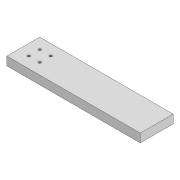
# Autodesk Inventor part: theplank
Saved by Autodesk Inventor 2020 (Build 240168000, 168)
## iProperties
Created: 2021-06-21
Part Number: theplank
Material: Generic
Document SubType Name: Modeling
Designer: Aidan Lee
Density: 1 g/cm^3
Appearance: Default
Author: Aidan Lee
Autodesk Inventor part; units mm, degrees
ref_plane "YZ Plane" through (0, 0, 0) normal (1, 0, 0) x (0, 1, 0)
ref_plane "XZ Plane" through (0, 0, 0) normal (0, 1, 0) x (-1, 0, 0)
ref_plane "XY Plane" through (0, 0, 0) normal (0, 0, 1) x (1, 0, 0)
sketch "Sketch1" plane through (0, 0, 0) normal (0, 1, 0) x (-1, 0, 0)
  line L0 (0, 0) -> (-280, 0)
  line L1 (-280, 0) -> (-280, -69)
  line L2 (-280, -69) -> (0, -69)
  line L3 (0, -69) -> (0, 0)
  dimension "d0" = 69
  dimension "d1" = 280
  constraints: 8 end point, 2 parallel, 1 horizontal, 1 perpendicular
  measures "d0" distance of L2.end L0.start
  measures "d1" distance of L1.end L2.end
extrude "Extrusion1" add sketch "Sketch1" along normal blind 18
sketch "Sketch2" plane through (0, 18, 0) normal (0, 1, 0) x (1, 0, 0)
  circle A0 centre (23, 23) radius 2.6
  circle A1 centre (46, 46) radius 2.6
  circle A2 centre (23, 46) radius 2.6
  circle A3 centre (46, 23) radius 2.6
  line L0 (46, 46) -> (23, 23)
  line L1 (23, 46) -> (46, 23)
  line L2 (0, 69) -> (0, 0) projected
  line L3 (0, 0) -> (280, 0) projected
  point P0 (34.5, 34.5)
  point P1 (34.5, 34.5)
  point P2 (0, 34.5)
  dimension "d4" = 5.2
  dimension "d5" = 5.2
  dimension "d6" = 5.2
  dimension "d7" = 5.2
  dimension "d8" = 23
  dimension "d9" = 23
  constraints: 4 centre point, 4 end point, 3 horizontal alignment, 3 midpoint, 2 vertical alignment, 1 perpendicular
  measures "d4" diameter of A0
  measures "d5" diameter of A3
  measures "d6" diameter of A1
  measures "d7" diameter of A2
  measures "d8" distance from line of L2 L0.end
  measures "d9" distance from line of L3 L0.end
extrude "Extrusion2" cut sketch "Sketch2" against normal through all
equation "\"d5\" = d4"
equation "\"d6\" = d4"
equation "\"d7\" = d4"
body "Solid1"
